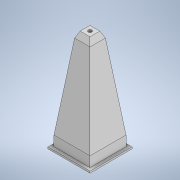
# Autodesk Inventor part: VRSPAD-144 illumination box
Saved by Autodesk Inventor 2022 (Build 260153000, 153)
## iProperties
Created: 2023-04-03
Part Number: VRSPAD-144 illumination box
Material: Generic
Document SubType Name: Modeling
Designer: William
Density: 1 g/cm^3
Appearance: Default
Author: William
Autodesk Inventor part; units mm, degrees
ref_plane "YZ Plane" through (0, 0, 0) normal (1, 0, 0) x (0, 1, 0)
ref_plane "XZ Plane" through (0, 0, 0) normal (0, 1, 0) x (-1, 0, 0)
ref_plane "XY Plane" through (0, 0, 0) normal (0, 0, 1) x (1, 0, 0)
sketch "Sketch1" plane through (0, 0, 0) normal (0, 1, 0) x (-1, 0, 0)
  line L0 (0, 0) -> (60, 0)
  line L1 (60, 0) -> (60, -60)
  line L2 (60, -60) -> (0, -60)
  line L3 (0, -60) -> (0, 0)
  point P0 (30, -60)
  point P1 (0, -30)
  dimension "d1" = 60
  constraints: 8 end point, 2 midpoint, 2 parallel, 2 perpendicular, 1 horizontal
  measures "d1" distance of L0.end L1.end
extrude "Extrusion1" add sketch "Sketch1" against normal blind 20
extrude "Extrusion2" add sketch "Sketch1" along normal blind 140 draft -7
shell "Shell1" thickness 1.2 removed faces 1 at (-20, -20, -20)
sketch "Sketch2" plane through (0, 140, 0) normal (0, 1, 0) x (1, 0, 0)
  line L0 (-17.1898, 42.8102) -> (-17.1898, 17.1898) projected
  line L1 (-42.8102, 42.8102) -> (-17.1898, 42.8102) projected
  line L2 (-42.8102, 17.1898) -> (-42.8102, 42.8102) projected
  line L3 (-17.1898, 17.1898) -> (-42.8102, 17.1898) projected
  circle A0 centre (-30, 30) radius 3
  point P0 (0, 0)
  point P1 (-30, 42.8102)
  point P2 (-42.8102, 30)
  dimension "d7" = 6
  constraints: 2 midpoint, 1 centre point, 1 horizontal alignment, 1 vertical alignment
  measures "d7" diameter of A0
extrude "Extrusion4" add sketch "Sketch2" along normal blind 10 draft -25 contours L0 L3 L2 L1 | A0
extrude "Extrusion3" cut sketch "Sketch2" along normal mid plane 25.4 contours A0
sketch "Sketch4" plane through (0, -20, 0) normal (0, -1, 0) x (1, 0, 0)
  line L0 (-65, -65) -> (5, -65)
  line L1 (5, -65) -> (5, 5)
  line L2 (5, 5) -> (-65, 5)
  line L3 (-65, 5) -> (-65, -65)
  line L4 (-58.8, -1.2) -> (-1.2, -1.2) projected
  line L5 (-1.2, -1.2) -> (-1.2, -58.8) projected
  line L6 (-58.8, -58.8) -> (-58.8, -1.2) projected
  line L7 (-1.2, -58.8) -> (-58.8, -58.8) projected
  point P0 (0, 0)
  point P1 (-30, 5)
  point P2 (-30, -1.2)
  point P3 (5, -30)
  point P4 (-1.2, -30)
  dimension "d16" = 70
  constraints: 8 end point, 4 midpoint, 2 parallel, 2 perpendicular, 1 horizontal, 1 horizontal alignment, 1 vertical alignment
  measures "d16" distance of L1.end L2.end
extrude "Extrusion6" add sketch "Sketch4" against normal blind 3
body "Solid1"
